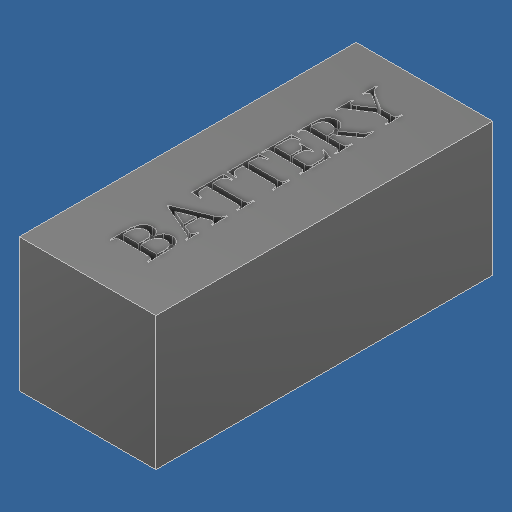
# Autodesk Inventor part: EBox-ArmBattery
Saved by Autodesk Inventor 2023 (Build 270158030, 158C)
## iProperties
Created: 2022-10-10
Part Number: EBox-ArmBattery
Material: Air
Document SubType Name: Modeling
Designer: Nebil
Density: 0.0012 g/cm^3
Appearance: Smooth - Black
Author: Nebil
Autodesk Inventor part; units mm, degrees
ref_plane "YZ Plane" through (0, 0, 0) normal (1, 0, 0) x (0, 1, 0)
ref_plane "XZ Plane" through (0, 0, 0) normal (0, 1, 0) x (-1, 0, 0)
ref_plane "XY Plane" through (0, 0, 0) normal (0, 0, 1) x (1, 0, 0)
sketch "Sketch1" plane through (0, 0, 0) normal (0, 1, 0) x (-1, 0, 0)
  line L0 (-22.5, -55.5) -> (22.5, -55.5)
  line L1 (22.5, -55.5) -> (22.5, 55.5)
  line L2 (22.5, 55.5) -> (-22.5, 55.5)
  line L3 (-22.5, 55.5) -> (-22.5, -55.5)
  line L4 (-22.5, -55.5) -> (22.5, 55.5) construction
  line L5 (22.5, -55.5) -> (-22.5, 55.5) construction
  point P0 (0, 0)
  dimension "d0" = 45
  dimension "d1" = 111
  constraints: 12 end point, 2 midpoint, 2 parallel, 1 horizontal, 1 perpendicular
  measures "d0" distance of L2.end L1.end
  measures "d1" distance of L1.end L0.end
extrude "Extrusion1" add sketch "Sketch1" along normal blind 44
sketch "Sketch2" plane through (0, 44, 0) normal (0, 1, 0) x (1, 0, 0)
  line L0 (-7.895, -52.325) -> (-7.895, 57.1567) construction
  line L1 (-7.895, 57.1567) -> (6.8329, 57.1567) construction
  line L2 (6.8329, 57.1567) -> (6.8329, -52.325) construction
  line L3 (6.8329, -52.325) -> (-7.895, -52.325) construction
  line L4 (-22.5, 55.5) -> (-22.5, -55.5) projected
  line L5 (22.5, -55.5) -> (22.5, 55.5) projected
  line L6 (-22.5, -55.5) -> (22.5, -55.5) projected
  spline S0 degree 2 poles (-0.5103, -32.9294) (-0.2301, -31.6116) (0.3924, -30.9579) knots 0 0 0 1 1 1
  spline S1 degree 2 poles (0.3924, -30.9579) (1.2432, -30.0449) (2.4883, -30.0449) knots 0 0 0 1 1 1
  spline S2 degree 2 poles (2.4883, -30.0449) (3.4325, -30.0449) (5.1653, -31.2485) (5.9642, -33.334) (5.9642, -35.4818) knots 0 0 0 1 2 3 3 3
  line L7 (5.9642, -35.4818) -> (5.9642, -41.479)
  line L8 (5.9642, -41.479) -> (5.6218, -41.479)
  line L9 (5.6218, -41.479) -> (5.6218, -41.0017)
  spline S3 degree 2 poles (5.6218, -41.0017) (5.6218, -40.2028) (5.1134, -39.8604) knots 0 0 0 1 1 1
  spline S4 degree 2 poles (5.1134, -39.8604) (4.7814, -39.6425) (3.7127, -39.6425) knots 0 0 0 1 1 1
  line L10 (3.7127, -39.6425) -> (-4.4842, -39.6425)
  spline S5 degree 2 poles (-4.4842, -39.6425) (-5.6671, -39.6425) (-5.9783, -39.9123) knots 0 0 0 1 1 1
  spline S6 degree 2 poles (-5.9783, -39.9123) (-6.3934, -40.2754) (-6.3934, -41.0017) knots 0 0 0 1 1 1
  line L11 (-6.3934, -41.0017) -> (-6.3934, -41.479)
  line L12 (-6.3934, -41.479) -> (-6.7358, -41.479)
  line L13 (-6.7358, -41.479) -> (-6.7358, -35.9902)
  spline S7 degree 2 poles (-6.7358, -35.9902) (-6.7358, -34.4546) (-6.5075, -33.5208) knots 0 0 0 1 1 1
  spline S8 degree 2 poles (-6.5075, -33.5208) (-6.1755, -32.12) (-4.4531, -30.6363) (-3.3429, -30.6363) knots 0 0 0 1 2 2 2
  spline S9 degree 2 poles (-3.3429, -30.6363) (-2.3883, -30.6363) (-0.8734, -31.7984) (-0.5103, -32.9294) knots 0 0 0 1 2 2 2
  spline S10 degree 2 poles (5.0511, -37.8475) (5.3002, -36.758) (5.3002, -35.6893) knots 0 0 0 1 1 1
  spline S11 degree 2 poles (5.3002, -35.6893) (5.3002, -33.9877) (3.7749, -32.1927) (2.6543, -32.1927) knots 0 0 0 1 2 2 2
  spline S12 degree 2 poles (2.6543, -32.1927) (1.9073, -32.1927) (0.548, -33.0227) (-0.2405, -34.8489) (-0.2405, -36.1874) knots 0 0 0 1 2 3 3 3
  spline S13 degree 2 poles (-0.2405, -36.1874) (-0.2405, -36.7684) (-0.199, -37.5985) (-0.1575, -37.8475) knots 0 0 0 1 2 2 2
  line L14 (-0.1575, -37.8475) -> (5.0511, -37.8475)
  spline S14 degree 2 poles (-1.0187, -37.8475) (-0.9461, -37.5051) (-0.8838, -36.6128) (-0.8838, -36.0732) knots 0 0 0 1 2 2 2
  spline S15 degree 2 poles (-0.8838, -36.0732) (-0.8838, -34.7036) (-1.4752, -33.3236) (-2.6996, -32.5973) (-3.4155, -32.5973) knots 0 0 0 1 2 3 3 3
  spline S16 degree 2 poles (-3.4155, -32.5973) (-4.5361, -32.5973) (-6.1132, -34.4131) (-6.1132, -36.1562) knots 0 0 0 1 2 2 2
  spline S17 degree 2 poles (-6.1132, -36.1562) (-6.1132, -37.1004) (-5.9057, -37.8475) knots 0 0 0 1 1 1
  line L15 (-5.9057, -37.8475) -> (-1.0187, -37.8475)
  line L16 (1.7205, -20.2086) -> (1.7205, -25.1475)
  line L17 (1.7205, -25.1475) -> (3.7127, -26.0087)
  spline S18 degree 2 poles (3.7127, -26.0087) (4.4597, -26.3303) (4.8229, -26.3303) knots 0 0 0 1 1 1
  spline S19 degree 2 poles (4.8229, -26.3303) (5.1134, -26.3303) (5.5596, -25.77) (5.6218, -24.857) knots 0 0 0 1 2 2 2
  line L18 (5.6218, -24.857) -> (5.9642, -24.857)
  line L19 (5.9642, -24.857) -> (5.9642, -28.862)
  line L20 (5.9642, -28.862) -> (5.6218, -28.862)
  spline S20 degree 2 poles (5.6218, -28.862) (5.4766, -28.0631) (5.2587, -27.8348) knots 0 0 0 1 1 1
  spline S21 degree 2 poles (5.2587, -27.8348) (4.8021, -27.3575) (3.4221, -26.7765) knots 0 0 0 1 1 1
  line L21 (3.4221, -26.7765) -> (-7.0263, -22.2941)
  line L22 (-7.0263, -22.2941) -> (-7.0263, -21.9621)
  line L23 (-7.0263, -21.9621) -> (3.5363, -17.542)
  spline S22 degree 2 poles (3.5363, -17.542) (4.8125, -17.0128) (5.5699, -16.1413) (5.6218, -15.3631) knots 0 0 0 1 2 2 2
  line L24 (5.6218, -15.3631) -> (5.9642, -15.3631)
  line L25 (5.9642, -15.3631) -> (5.9642, -20.3746)
  line L26 (5.9642, -20.3746) -> (5.6218, -20.3746)
  spline S23 degree 2 poles (5.6218, -20.3746) (5.5803, -19.6172) (5.1549, -19.0776) (4.8436, -19.0776) knots 0 0 0 1 2 2 2
  spline S24 degree 2 poles (4.8436, -19.0776) (4.4286, -19.0776) (3.5363, -19.4512) knots 0 0 0 1 1 1
  line L27 (3.5363, -19.4512) -> (1.7205, -20.2086)
  line L28 (1.0253, -20.4991) -> (-4.1107, -22.6365)
  line L29 (-4.1107, -22.6365) -> (1.0253, -24.8466)
  line L30 (1.0253, -24.8466) -> (1.0253, -20.4991)
  line L31 (-6.7358, -4.0638) -> (-3.7579, -3.9289)
  line L32 (-3.7579, -3.9289) -> (-3.7579, -4.2817)
  spline S25 degree 2 poles (-3.7579, -4.2817) (-4.5361, -4.3855) (-4.8785, -4.5619) knots 0 0 0 1 1 1
  spline S26 degree 2 poles (-4.8785, -4.5619) (-5.4181, -4.8524) (-5.9368, -5.8173) (-5.9368, -6.6059) knots 0 0 0 1 2 2 2
  line L33 (-5.9368, -6.6059) -> (-5.9368, -8.3905)
  line L34 (-5.9368, -8.3905) -> (3.7645, -8.3905)
  spline S27 degree 2 poles (3.7645, -8.3905) (4.937, -8.3905) (5.2275, -8.1415) knots 0 0 0 1 1 1
  spline S28 degree 2 poles (5.2275, -8.1415) (5.6218, -7.7784) (5.6218, -7.0417) knots 0 0 0 1 1 1
  line L35 (5.6218, -7.0417) -> (5.6218, -6.6059)
  line L36 (5.6218, -6.6059) -> (5.9642, -6.6059)
  line L37 (5.9642, -6.6059) -> (5.9642, -11.9806)
  line L38 (5.9642, -11.9806) -> (5.6218, -11.9806)
  line L39 (5.6218, -11.9806) -> (5.6218, -11.5344)
  spline S29 degree 2 poles (5.6218, -11.5344) (5.6218, -10.7251) (5.1342, -10.3931) knots 0 0 0 1 1 1
  spline S30 degree 2 poles (5.1342, -10.3931) (4.8333, -10.1856) (3.7645, -10.1856) knots 0 0 0 1 1 1
  line L40 (3.7645, -10.1856) -> (-5.9368, -10.1856)
  line L41 (-5.9368, -10.1856) -> (-5.9368, -11.7108)
  spline S31 degree 2 poles (-5.9368, -11.7108) (-5.9368, -12.6031) (-5.802, -12.9767) knots 0 0 0 1 1 1
  spline S32 degree 2 poles (-5.802, -12.9767) (-5.6256, -13.4643) (-4.6191, -14.1491) (-3.7579, -14.2218) knots 0 0 0 1 2 2 2
  line L42 (-3.7579, -14.2218) -> (-3.7579, -14.5745)
  line L43 (-3.7579, -14.5745) -> (-6.7358, -14.4293)
  line L44 (-6.7358, -14.4293) -> (-6.7358, -4.0638)
  line L45 (-6.7358, 7.6505) -> (-3.7579, 7.7854)
  line L46 (-3.7579, 7.7854) -> (-3.7579, 7.4326)
  spline S33 degree 2 poles (-3.7579, 7.4326) (-4.5361, 7.3288) (-4.8785, 7.1524) knots 0 0 0 1 1 1
  spline S34 degree 2 poles (-4.8785, 7.1524) (-5.4181, 6.8619) (-5.9368, 5.897) (-5.9368, 5.1084) knots 0 0 0 1 2 2 2
  line L47 (-5.9368, 5.1084) -> (-5.9368, 3.3238)
  line L48 (-5.9368, 3.3238) -> (3.7645, 3.3238)
  spline S35 degree 2 poles (3.7645, 3.3238) (4.937, 3.3238) (5.2275, 3.5728) knots 0 0 0 1 1 1
  spline S36 degree 2 poles (5.2275, 3.5728) (5.6218, 3.9359) (5.6218, 4.6726) knots 0 0 0 1 1 1
  line L49 (5.6218, 4.6726) -> (5.6218, 5.1084)
  line L50 (5.6218, 5.1084) -> (5.9642, 5.1084)
  line L51 (5.9642, 5.1084) -> (5.9642, -0.2663)
  line L52 (5.9642, -0.2663) -> (5.6218, -0.2663)
  line L53 (5.6218, -0.2663) -> (5.6218, 0.1799)
  spline S37 degree 2 poles (5.6218, 0.1799) (5.6218, 0.9892) (5.1342, 1.3212) knots 0 0 0 1 1 1
  spline S38 degree 2 poles (5.1342, 1.3212) (4.8333, 1.5287) (3.7645, 1.5287) knots 0 0 0 1 1 1
  line L54 (3.7645, 1.5287) -> (-5.9368, 1.5287)
  line L55 (-5.9368, 1.5287) -> (-5.9368, 0.0035)
  spline S39 degree 2 poles (-5.9368, 0.0035) (-5.9368, -0.8888) (-5.802, -1.2624) knots 0 0 0 1 1 1
  spline S40 degree 2 poles (-5.802, -1.2624) (-5.6256, -1.75) (-4.6191, -2.4348) (-3.7579, -2.5075) knots 0 0 0 1 2 2 2
  line L56 (-3.7579, -2.5075) -> (-3.7579, -2.8602)
  line L57 (-3.7579, -2.8602) -> (-6.7358, -2.715)
  line L58 (-6.7358, -2.715) -> (-6.7358, 7.6505)
  line L59 (-6.0406, 12.2781) -> (-1.0291, 12.2781)
  line L60 (-1.0291, 12.2781) -> (-1.0291, 15.0692)
  spline S41 degree 2 poles (-1.0291, 15.0692) (-1.0291, 16.1586) (-1.3611, 16.5218) knots 0 0 0 1 1 1
  spline S42 degree 2 poles (-1.3611, 16.5218) (-1.7865, 17.0198) (-2.876, 17.0717) knots 0 0 0 1 1 1
  line L61 (-2.876, 17.0717) -> (-2.876, 17.4141)
  line L62 (-2.876, 17.4141) -> (1.5545, 17.4141)
  line L63 (1.5545, 17.4141) -> (1.5545, 17.0717)
  spline S43 degree 2 poles (1.5545, 17.0717) (0.631, 16.9368) (0.3717, 16.8123) knots 0 0 0 1 1 1
  spline S44 degree 2 poles (0.3717, 16.8123) (0.0396, 16.6359) (-0.3339, 15.8681) (-0.3339, 15.0692) knots 0 0 0 1 2 2 2
  line L64 (-0.3339, 15.0692) -> (-0.3339, 12.2781)
  line L65 (-0.3339, 12.2781) -> (3.8476, 12.2781)
  spline S45 degree 2 poles (3.8476, 12.2781) (4.688, 12.2781) (5.0511, 12.4233) (5.269, 12.8073) (5.269, 13.326) knots 0 0 0 1 2 3 3 3
  line L66 (5.269, 13.326) -> (5.269, 15.4842)
  spline S46 degree 2 poles (5.269, 15.4842) (5.269, 16.5633) (4.9681, 17.5386) (4.5324, 17.9848) knots 0 0 0 1 2 2 2
  spline S47 degree 2 poles (4.5324, 17.9848) (3.9513, 18.5658) (2.7788, 19.178) knots 0 0 0 1 1 1
  line L67 (2.7788, 19.178) -> (2.7788, 19.5515)
  line L68 (2.7788, 19.5515) -> (5.9642, 18.4517)
  line L69 (5.9642, 18.4517) -> (5.9642, 8.6673)
  line L70 (5.9642, 8.6673) -> (5.6218, 8.6673)
  line L71 (5.6218, 8.6673) -> (5.6218, 9.1135)
  spline S48 degree 2 poles (5.6218, 9.1135) (5.6218, 9.57) (5.4039, 9.9643) knots 0 0 0 1 1 1
  spline S49 degree 2 poles (5.4039, 9.9643) (5.2483, 10.2652) (4.6465, 10.4831) (3.7127, 10.4831) knots 0 0 0 1 2 2 2
  line L72 (3.7127, 10.4831) -> (-4.5257, 10.4831)
  spline S50 degree 2 poles (-4.5257, 10.4831) (-5.7397, 10.4831) (-6.0199, 10.2444) knots 0 0 0 1 1 1
  spline S51 degree 2 poles (-6.0199, 10.2444) (-6.3934, 9.902) (-6.3934, 9.1135) knots 0 0 0 1 1 1
  line L73 (-6.3934, 9.1135) -> (-6.3934, 8.6673)
  line L74 (-6.3934, 8.6673) -> (-6.7358, 8.6673)
  line L75 (-6.7358, 8.6673) -> (-6.7358, 18.4621)
  line L76 (-6.7358, 18.4621) -> (-3.9447, 18.597)
  line L77 (-3.9447, 18.597) -> (-3.9447, 18.2338)
  spline S52 degree 2 poles (-3.9447, 18.2338) (-4.9511, 18.0367) (-5.6982, 17.5594) (-5.8953, 17.0925) knots 0 0 0 1 2 2 2
  spline S53 degree 2 poles (-5.8953, 17.0925) (-6.0406, 16.7189) (-6.0406, 15.7644) knots 0 0 0 1 1 1
  line L78 (-6.0406, 15.7644) -> (-6.0406, 12.2781)
  line L79 (5.9642, 32.9571) -> (5.9642, 29.5642)
  line L80 (5.9642, 29.5642) -> (0.0293, 25.2582)
  spline S54 degree 2 poles (0.0293, 25.2582) (0.05, 24.7809) (0.05, 24.4904) knots 0 0 0 1 1 1
  spline S55 degree 2 poles (0.05, 24.4904) (0.05, 24.3659) (0.0396, 24.0858) (0.0293, 23.9405) knots 0 0 0 1 2 2 2
  line L81 (0.0293, 23.9405) -> (3.7127, 23.9405)
  spline S56 degree 2 poles (3.7127, 23.9405) (4.9163, 23.9405) (5.2068, 24.1999) knots 0 0 0 1 1 1
  spline S57 degree 2 poles (5.2068, 24.1999) (5.6218, 24.5527) (5.6218, 25.2582) knots 0 0 0 1 1 1
  line L82 (5.6218, 25.2582) -> (5.6218, 25.7563)
  line L83 (5.6218, 25.7563) -> (5.9642, 25.7563)
  line L84 (5.9642, 25.7563) -> (5.9642, 20.3297)
  line L85 (5.9642, 20.3297) -> (5.6218, 20.3297)
  line L86 (5.6218, 20.3297) -> (5.6218, 20.807)
  spline S58 degree 2 poles (5.6218, 20.807) (5.6218, 21.6059) (5.0926, 21.9483) knots 0 0 0 1 1 1
  spline S59 degree 2 poles (5.0926, 21.9483) (4.8021, 22.1455) (3.7127, 22.1455) knots 0 0 0 1 1 1
  line L87 (3.7127, 22.1455) -> (-4.4842, 22.1455)
  spline S60 degree 2 poles (-4.4842, 22.1455) (-5.6878, 22.1455) (-5.9783, 21.8861) knots 0 0 0 1 1 1
  spline S61 degree 2 poles (-5.9783, 21.8861) (-6.3934, 21.5229) (-6.3934, 20.807) knots 0 0 0 1 1 1
  line L88 (-6.3934, 20.807) -> (-6.3934, 20.3297)
  line L89 (-6.3934, 20.3297) -> (-6.7358, 20.3297)
  line L90 (-6.7358, 20.3297) -> (-6.7358, 24.947)
  spline S62 degree 2 poles (-6.7358, 24.947) (-6.7358, 26.9702) (-6.1444, 28.8898) (-4.5672, 30.2282) (-3.4674, 30.2282) knots 0 0 0 1 2 3 3 3
  spline S63 degree 2 poles (-3.4674, 30.2282) (-2.2949, 30.2282) (-0.5725, 28.703) (-0.2198, 27.0947) knots 0 0 0 1 2 2 2
  line L91 (-0.2198, 27.0947) -> (3.4221, 29.7302)
  spline S64 degree 2 poles (3.4221, 29.7302) (4.6776, 30.6329) (5.5077, 31.9195) (5.6218, 32.9571) knots 0 0 0 1 2 2 2
  line L92 (5.6218, 32.9571) -> (5.9642, 32.9571)
  spline S65 degree 2 poles (-0.5622, 23.9405) (-0.5622, 24.1169) (-0.5518, 24.3763) (-0.5518, 24.4593) knots 0 0 0 1 2 2 2
  spline S66 degree 2 poles (-0.5518, 24.4593) (-0.5518, 26.2543) (-2.1289, 28.0805) (-3.3429, 28.0805) knots 0 0 0 1 2 2 2
  spline S67 degree 2 poles (-3.3429, 28.0805) (-4.5361, 28.0805) (-6.0199, 26.6071) (-6.0199, 25.3931) knots 0 0 0 1 2 2 2
  spline S68 degree 2 poles (-6.0199, 25.3931) (-6.0199, 24.8536) (-5.8435, 23.9405) knots 0 0 0 1 1 1
  line L93 (-5.8435, 23.9405) -> (-0.5622, 23.9405)
  line L94 (-6.7358, 41.9218) -> (-6.7358, 46.3626)
  line L95 (-6.7358, 46.3626) -> (-6.3934, 46.3626)
  line L96 (-6.3934, 46.3626) -> (-6.3934, 46.1136)
  spline S69 degree 2 poles (-6.3934, 46.1136) (-6.3934, 45.875) (-5.9576, 44.9412) (-5.1483, 44.1733) (-4.2456, 43.6027) knots 0 0 0 1 2 3 3 3
  line L97 (-4.2456, 43.6027) -> (0.5688, 40.5418)
  line L98 (0.5688, 40.5418) -> (3.7645, 40.5418)
  spline S70 degree 2 poles (3.7645, 40.5418) (4.937, 40.5418) (5.2275, 40.8012) knots 0 0 0 1 1 1
  spline S71 degree 2 poles (5.2275, 40.8012) (5.6218, 41.154) (5.6218, 41.9218) knots 0 0 0 1 1 1
  line L99 (5.6218, 41.9218) -> (5.6218, 42.3368)
  line L100 (5.6218, 42.3368) -> (5.9642, 42.3368)
  line L101 (5.9642, 42.3368) -> (5.9642, 36.9518)
  line L102 (5.9642, 36.9518) -> (5.6218, 36.9518)
  line L103 (5.6218, 36.9518) -> (5.6218, 37.3979)
  spline S72 degree 2 poles (5.6218, 37.3979) (5.6218, 38.2072) (5.1342, 38.5393) knots 0 0 0 1 1 1
  spline S73 degree 2 poles (5.1342, 38.5393) (4.8333, 38.7468) (3.7645, 38.7468) knots 0 0 0 1 1 1
  line L104 (3.7645, 38.7468) -> (0.7659, 38.7468)
  line L105 (0.7659, 38.7468) -> (-4.5672, 35.2709)
  spline S74 degree 2 poles (-4.5672, 35.2709) (-5.5011, 34.6483) (-5.968, 34.2126) (-6.3, 33.5174) knots 0 0 0 1 2 2 2
  spline S75 degree 2 poles (-6.3, 33.5174) (-6.3934, 33.3306) (-6.3934, 32.9778) knots 0 0 0 1 1 1
  line L106 (-6.3934, 32.9778) -> (-6.7358, 32.9778)
  line L107 (-6.7358, 32.9778) -> (-6.7358, 38.394)
  line L108 (-6.7358, 38.394) -> (-6.3934, 38.394)
  line L109 (-6.3934, 38.394) -> (-6.3934, 38.1139)
  spline S76 degree 2 poles (-6.3934, 38.1139) (-6.3934, 37.6781) (-5.9783, 36.9414) (-5.5633, 36.9414) knots 0 0 0 1 2 2 2
  spline S77 degree 2 poles (-5.5633, 36.9414) (-5.2313, 36.9414) (-4.3493, 37.5121) knots 0 0 0 1 1 1
  line L110 (-4.3493, 37.5121) -> (-0.2509, 40.1579)
  line L111 (-0.2509, 40.1579) -> (-4.173, 42.6481)
  spline S78 degree 2 poles (-4.173, 42.6481) (-5.0549, 43.2084) (-5.4803, 43.2084) knots 0 0 0 1 1 1
  spline S79 degree 2 poles (-5.4803, 43.2084) (-5.7501, 43.2084) (-6.1547, 42.9386) (-6.3934, 42.4302) (-6.3934, 41.9218) knots 0 0 0 1 2 3 3 3
  line L112 (-6.3934, 41.9218) -> (-6.7358, 41.9218)
  point P0 (0, 0)
  dimension "d4" = 14.605
  dimension "d6" = 3.175
  constraints: 2 other
  measures "d4" distance between parallel lines of L4 L0
  measures "d6" distance between parallel lines of L6 L3
emboss "Emboss1" sketch "Sketch2" operation cut depth 2.54 direction (0, -1, 0)
body "Solid1"
